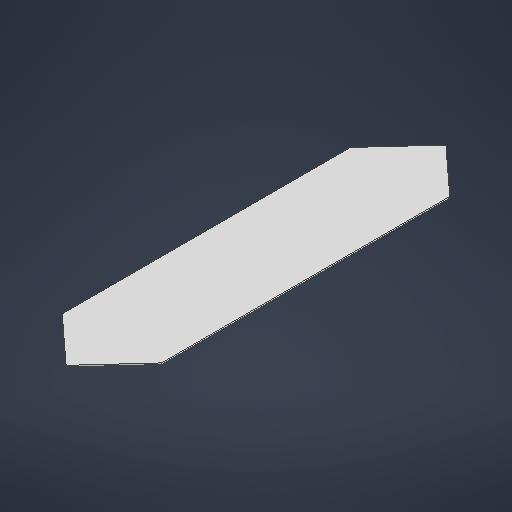
# Autodesk Inventor part: g
Saved by Autodesk Inventor 2027 (Build 310192000, 192)
## iProperties
Created: 2026-02-05
Part Number: g
Material: Generic
Document SubType Name: Modeling
Designer: Joefi
Density: 1 g/cm^3
Appearance: Default
Author: Joefi
Autodesk Inventor part; units mm, degrees
ref_plane "YZ Plane" through (0, 0, 0) normal (1, 0, 0) x (0, 1, 0)
ref_plane "XZ Plane" through (0, 0, 0) normal (0, 1, 0) x (-1, 0, 0)
ref_plane "XY Plane" through (0, 0, 0) normal (0, 0, 1) x (1, 0, 0)
sketch "Sketch1" plane through (0, 0, 0) normal (0, 1, 0) x (-1, 0, 0)
  line L0 (13, -39.6468) -> (13, 41.6738)
  line L1 (13, 41.6738) -> (-0.1234, 53.6991)
  line L2 (-0.1234, 53.6991) -> (-13, 39.6468)
  line L3 (-13, 39.6468) -> (-13, -41.6738)
  line L4 (-13, -41.6738) -> (0.1234, -53.6991)
  line L5 (0.1234, -53.6991) -> (13, -39.6468)
  line L6 (-9.6864, 40.3026) -> (-3.378, 47.187)
  arc A0 (3.6864, 47.4955) -> (-3.378, 47.187) centre (0.3084, 43.8091) ccw
  line L7 (3.6864, 47.4955) -> (9.378, 42.2801)
  arc A1 (11, 38.5937) -> (9.378, 42.2801) centre (6, 38.5937) ccw
  line L8 (11, 38.5937) -> (11, -36.9246)
  arc A2 (9.6864, -40.3026) -> (11, -36.9246) centre (6, -36.9246) ccw
  line L9 (9.6864, -40.3026) -> (3.378, -47.187)
  arc A3 (-3.6864, -47.4955) -> (3.378, -47.187) centre (-0.3084, -43.8091) ccw
  line L10 (-3.6864, -47.4955) -> (-9.378, -42.2801)
  arc A4 (-11, -38.5937) -> (-9.378, -42.2801) centre (-6, -38.5937) ccw
  line L11 (-11, -38.5937) -> (-11, 36.9246)
  arc A5 (-9.6864, 40.3026) -> (-11, 36.9246) centre (-6, 36.9246) ccw
  line L12 (12.8, -39.569) -> (0.111, -53.4166)
  line L13 (0.111, -53.4166) -> (-12.8, -41.5858)
  line L14 (-12.8, -41.5858) -> (-12.8, 39.569)
  line L15 (-12.8, 39.569) -> (-0.111, 53.4166)
  point P0 (0, 0)
  point P1 (0, 0)
  constraints: 32 end point, 12 point on circle, 6 centre point, 3 other
extrude "Extrusion1" add sketch "Sketch1" along normal blind 0.4 contours L5 L4 L3 L2 L1 L0 | L6 A0 L7 A1 L8 A2 L9 A3 L10 A4 L11 A5
body "Solid1"
